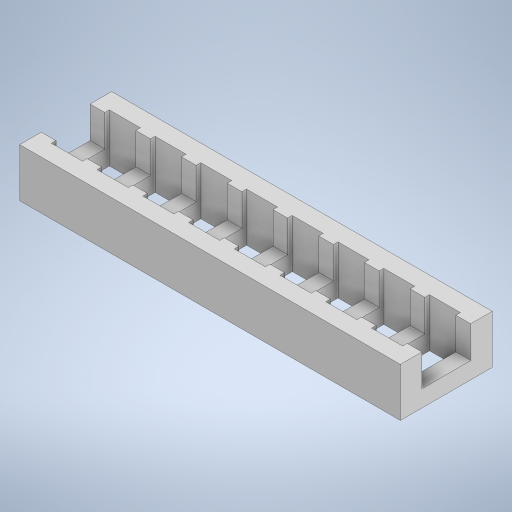
# Autodesk Inventor part: LatchHolder
Saved by Autodesk Inventor 2024 (Build 280153000, 153)
## iProperties
Created: 2024-03-21
Part Number: LatchHolder
Material: Generic
Document SubType Name: Modeling
Designer: gcter
Density: 1 g/cm^3
Appearance: Default
Author: gcter
Autodesk Inventor part; units mm, degrees
ref_plane "YZ Plane" through (0, 0, 0) normal (1, 0, 0) x (0, 1, 0)
ref_plane "XZ Plane" through (0, 0, 0) normal (0, 1, 0) x (-1, 0, 0)
ref_plane "XY Plane" through (0, 0, 0) normal (0, 0, 1) x (1, 0, 0)
sketch "Sketch4" plane through (0, 0, 0) normal (0, 1, 0) x (-1, 0, 0)
  line L0 (0, -20.574) -> (0, -15.748)
  line L1 (0, -15.748) -> (-3.302, -15.748)
  line L2 (-3.302, -15.748) -> (-3.302, -16.764)
  line L3 (-3.302, -16.764) -> (-10.2362, -16.764)
  line L4 (-10.2362, -16.764) -> (-10.2362, -20.574)
  line L5 (-10.2362, -20.574) -> (0, -20.574)
  line L6 (0, 0) -> (0, -4.826)
  line L7 (0, -4.826) -> (-3.302, -4.826)
  line L8 (-3.302, -4.826) -> (-3.302, -3.81)
  line L9 (-3.302, -3.81) -> (-10.2362, -3.81)
  line L10 (-10.2362, -3.81) -> (-10.2362, 0)
  line L11 (-10.2362, 0) -> (0, 0)
  dimension "d22" = 3.302
  dimension "d23" = 1.016
  dimension "d24" = 1.016
  dimension "d25" = 6.9342
  dimension "d26" = 3.81
  dimension "d27" = 20.574
  dimension "d28" = 3.81
  constraints: 24 end point, 9 perpendicular, 3 collinear, 3 vertical
  measures "d22" distance between parallel lines of L0 L2
  measures "d23" distance between parallel lines of L1 L3
  measures "d24" distance between parallel lines of L9 L7
  measures "d25" distance between parallel lines of L4 L2
  measures "d26" distance between parallel lines of L3 L5
  measures "d27" distance between parallel lines of L11 L5
  measures "d28" distance between parallel lines of L11 L9
extrude "Extrusion4" add sketch "Sketch4" along normal blind 10.8712
sketch "Sketch5" plane through (0, 0, 0) normal (0, -1, 0) x (1, 0, 0)
  line L0 (0, -15.748) -> (3.302, -15.748)
  line L1 (3.302, -15.748) -> (3.302, -4.826)
  line L2 (3.302, -4.826) -> (0, -4.826)
  line L3 (0, -4.826) -> (0, -15.748)
  line L4 (3.302, -4.826) -> (0, -4.826) projected
  line L5 (0, -15.748) -> (3.302, -15.748) projected
  line L6 (0, -20.574) -> (0, -15.748) projected
  line L7 (3.302, -15.748) -> (3.302, -16.764) projected
  point P0 (0, 0)
  constraints: 8 end point, 4 collinear, 2 parallel, 1 horizontal, 1 perpendicular
extrude "Extrusion5" add sketch "Sketch5" against normal blind 3.7592
pattern_linear "Rectangular Pattern2" count 8 spacing 10.2362 along (1, 0, 0) of "Extrusion4", "Extrusion5"
sketch "Sketch6" plane through (81.8896, 0, -16.764) normal (1, 0, 0) x (0, 0, -1)
  line L0 (3.81, 0) -> (-16.764, 0) projected
  line L1 (3.81, 10.8712) -> (-1.016, 10.8712) projected
  line L2 (3.81, 0) -> (3.81, 10.8712)
  line L3 (3.81, 10.8712) -> (-1.016, 10.8712)
  line L4 (-11.938, 3.7592) -> (-1.016, 3.7592) projected
  line L5 (-1.016, 10.8712) -> (-1.016, 3.7592)
  line L6 (-1.016, 3.7592) -> (-11.938, 3.7592)
  line L7 (-11.938, 3.7592) -> (-11.938, 10.8712) projected
  line L8 (-11.938, 3.7592) -> (-11.938, 10.8712)
  line L9 (-16.764, 0) -> (-16.764, 10.8712) projected
  line L10 (-11.938, 10.8712) -> (-16.764, 10.8712)
  line L11 (-16.764, 10.8712) -> (-16.764, 0)
  line L12 (3.81, 0) -> (-16.764, 0)
  constraints: 16 end point, 6 perpendicular, 1 collinear, 1 vertical
extrude "Extrusion6" add sketch "Sketch6" along normal blind 3.302
body "Solid2"
